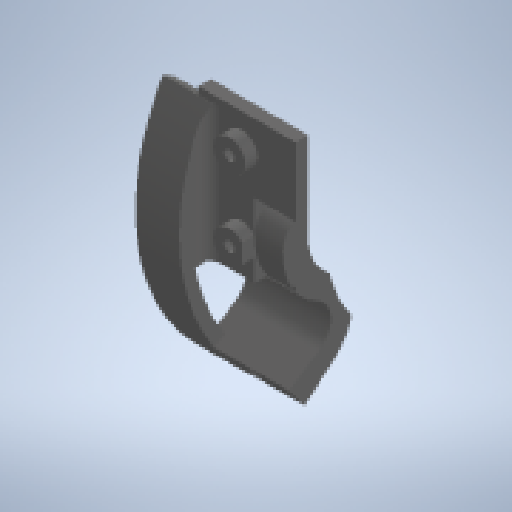
# Autodesk Inventor part: cover_back_right
Saved by Autodesk Inventor 2024.1 (Build 281209000, 209)
## iProperties
Created: 2025-01-10
Part Number: cover_back_right
Material: 一般
Document SubType Name: Modeling
Designer: hibik
Density: 1 g/cm^3
Appearance: 既定
Author: hibik
Autodesk Inventor part; units mm, degrees
ref_plane "YZ Plane" through (0, 0, 0) normal (1, 0, 0) x (0, 1, 0)
ref_plane "XZ Plane" through (0, 0, 0) normal (0, 1, 0) x (-1, 0, 0)
sketch "スケッチ1" plane through (0, 0, 0) normal (0, 0, 1) x (1, 0, 0)
  line L0 (10.5, 6.25) -> (-10.5, 6.25) construction
  line L1 (-10.5, 6.25) -> (-10.5, -6.25) construction
  line L2 (-10.5, -6.25) -> (10.5, -6.25) construction
  line L3 (10.5, -6.25) -> (10.5, 6.25) construction
  line L4 (10.5, 6.25) -> (-10.5, -6.25) construction
  line L5 (-10.5, 6.25) -> (10.5, -6.25) construction
  line L6 (-15.9, 11.28) -> (-2, 11.28)
  line L7 (-2, 11.28) -> (-2, -11.28)
  line L8 (-2, -11.28) -> (-15.9, -11.28)
  line L9 (-15.9, -11.28) -> (-15.9, 11.28)
  circle A0 centre (-10.5, 6.25) radius 0.85
  circle A1 centre (-10.5, -6.25) radius 0.85
  point P0 (0, 0)
  dimension "d0" = 21
  dimension "d1" = 12.5
  dimension "d2" = 2
  dimension "d3" = 15.9
  dimension "d4" = 5.03
  dimension "d5" = 5.03
  dimension "d7" = 1.7
  dimension "d8" = 1.7
  constraints: 20 end point, 4 parallel, 2 centre point, 2 coincident, 2 horizontal, 2 midpoint, 2 perpendicular
  measures "d0" distance of L0.start L0.end
  measures "d1" distance of L0.end L1.end
  measures "d2" distance from line of point (0, 0) L7
  measures "d3" distance from line of point (0, 0) L9
  measures "d4" distance between parallel lines of L6 L0
  measures "d5" distance between parallel lines of L8 L2
  measures "d7" diameter of A0
  measures "d8" diameter of A1
extrude "押し出し1" add sketch "スケッチ1" along normal blind 2
sketch "スケッチ2" plane through (0, 0, 2) normal (0, 0, 1) x (1, 0, 0)
  circle A0 centre (-10.5, 6.25) radius 0.85 projected
  circle A1 centre (-10.5, -6.25) radius 0.85 projected
  circle A2 centre (-10.5, 6.25) radius 2.5
  circle A3 centre (-10.5, -6.25) radius 2.5
  point P0 (0, 0)
  dimension "d11" = 5
  dimension "d12" = 5
  constraints: 2 centre point, 2 coincident
  measures "d11" diameter of A2
  measures "d12" diameter of A3
extrude "押し出し2" add sketch "スケッチ2" along normal blind 2
sketch "スケッチ3" plane through (-15.9, -11.28, 0) normal (-1, 0, 0) x (0, 0, 1)
  circle A0 centre (-26.25, 5.08) radius 26.25
  circle A1 centre (-26.25, 5.08) radius 30.75
  circle A2 centre (-26.25, 5.08) radius 32.75
  line L0 (6.5, 30) -> (6.5, 0) construction
  line L1 (4, 15.03) -> (4, 20.03) projected
  line L2 (-26.25, 5.08) -> (2.1123, 21.455)
  line L3 (-26.25, 5.08) -> (-9.875, -23.2823)
  line L4 (0, 22.56) -> (0, 0) projected
  line L5 (4, 18.38) -> (4, 16.68) projected
  line L6 (-72.1, 11.28) -> (19.6, 11.28) projected
  point P0 (0, 11.28)
  point P1 (0, 5.08)
  point P2 (0.3803, 20.455)
  point P3 (-10.875, -21.5503)
  point P4 (4, 17.53)
  dimension "d15" = 52.5
  dimension "d16" = 2.5
  dimension "d17" = 2
  dimension "d18" = 90
  dimension "d36" = 12.45
  dimension "d37" = 30
  constraints: 6 end point, 3 centre point, 2 coincident, 2 point on circle, 2 tangent, 1 horizontal alignment, 1 midpoint, 1 vertical
  measures "d15" diameter of A0
  measures "d16" distance between parallel lines of L1 L0
  measures "d17" radial gap between concentric circles of A2 A1
  measures "d18" angle of L3 L2
  measures "d36" vertical distance of point (4, 17.53) A0.centre
  measures "d37" angle of L6 L2
extrude "押し出し3" add sketch "スケッチ3" along normal blind 7 contours A1 L6 A2 L3 | A1 L2 A2 L6 picked at (5.3708, 0.6792) picked at (4.1065, 13.0583)
sketch "スケッチ5" plane through (0, 0, 0) normal (0, 0, -1) x (-1, 0, 0)
  line L0 (2, -11.28) -> (2, 11.28) projected
  line L1 (15.9, -11.28) -> (2, -11.28) projected
  line L2 (2, -4.75) -> (8.5, -4.75)
  line L3 (8.5, -4.75) -> (8.5, -11.28)
  line L4 (8.5, -11.28) -> (2, -11.28)
  line L5 (2, -11.28) -> (2, -4.75)
  line L6 (2, 11.28) -> (15.9, 11.28) projected
  circle A0 centre (10.5, 6.25) radius 0.85 projected
  circle A1 centre (10.5, -6.25) radius 2
  circle A2 centre (10.5, -6.25) radius 0.85 projected
  point P0 (0, 0)
  dimension "d26" = 11
  dimension "d27" = 4
  constraints: 8 end point, 2 parallel, 2 point on line, 1 centre point, 1 concentric, 1 horizontal, 1 perpendicular, 1 tangent
  measures "d26" distance from line of L2 A0.centre
  measures "d27" diameter of A1
extrude "押し出し5" cut sketch "スケッチ5" against normal through all contours L0 L2 L3 L1
sketch "スケッチ6" plane through (-2, 11.28, 2) normal (1, 0, 0) x (0, 0, -1)
  circle A0 centre (4, -16.03) radius 4
  line L0 (0, -16.03) -> (0, 0) projected
  line L1 (0, -16.03) -> (2, -16.03) projected
  line L2 (2, -16.03) -> (2, 0) projected
  line L3 (2, 0) -> (0, 0) projected
  line L4 (0, -16.03) -> (0, 0) projected
  circle A1 centre (4, -16.03) radius 6.5
  point P0 (2, -11.28)
  point P1 (2, -9.8453)
  point P2 (0, -10.9065)
  point P3 (0, -16.03)
  point P4 (2, -12.5659)
  dimension "d30" = 8
  dimension "d31" = 13
  constraints: 2 centre point, 1 coincident, 1 horizontal alignment, 1 tangent
  measures "d30" diameter of A0
  measures "d31" diameter of A1
extrude "押し出し6" cut sketch "スケッチ6" against normal up to surface (6.5 mm away) contours L0 A1 L2 A0 picked at (1.1078, -12.1766)
sketch "スケッチ7" plane through (-2, -4.75, 0) normal (1, 0, 0) x (0, 0, -1)
  circle A0 centre (2, 0) radius 4
  arc A1 (0, 3.4641) -> (-2, 0) centre (2, 0) ccw projected
  line L0 (-2, 0) -> (0, 0) projected
  line L1 (-2, 0) -> (6, 0)
  line L2 (2, 0) -> (2, 4)
  point P0 (0, 4.75)
  point P1 (-2, 0)
  constraints: 4 end point, 2 concentric, 2 point on circle, 1 centre point, 1 midpoint, 1 vertical
extrude "押し出し7" add sketch "スケッチ7" against normal up to surface (13.9 mm away) contours L2 L1 L0 A0
sketch "スケッチ8" plane through (-15.9, 11.28, 0) normal (-1, 0, 0) x (0, 0, 1)
  line L0 (2.1123, -1.105) -> (0.3803, -2.105) projected
  arc A0 (-10.875, -44.1103) -> (0.3803, -2.105) centre (-26.25, -17.48) ccw projected
  line L1 (-10.875, -44.1103) -> (-9.875, -45.8423) projected
  arc A1 (-9.875, -45.8423) -> (2.1123, -1.105) centre (-26.25, -17.48) ccw projected
  line L2 (0, -22.56) -> (2, -22.56) projected
  line L3 (0, -22.56) -> (-26.25, -17.48) construction
  line L4 (0, -22.56) -> (3.9399, -23.3225)
  line L5 (2, -5.335) -> (2, -22.56) projected
  arc A2 (2, -5.335) -> (0.3803, -2.105) centre (-26.25, -17.48) ccw projected
  line L6 (0.3803, -2.105) -> (2, -1.1699) projected
  line L7 (2, 0) -> (2, -1.1699) projected
  line L8 (0, 0) -> (2, 0) projected
  line L9 (0, 0) -> (0, -12.5659) projected
  arc A3 (0, -12.5659) -> (-2, -12.03) centre (-2, -16.03) ccw projected
  line L10 (-2, -16.03) -> (-2, -12.03) projected
  line L11 (0, -16.03) -> (-2, -16.03) projected
  line L12 (0, -16.03) -> (0, -22.56) projected
  line L13 (0, -22.56) -> (2, -22.56) projected
  point P0 (0, -11.28)
  point P1 (2, -1.1699)
  constraints: 4 end point, 1 coincident, 1 collinear, 1 point on circle
extrude "押し出し8" add sketch "スケッチ8" along normal blind 1.5 contours L0 A0 L5 L2 L12 L11 L10 A3 L9 L8 L7 | A0 L4 L2 L5
fillet "フィレット1" radius 2 2 edges at (-15.9, -2.6675, 2) (-15.9, 8.0276, 2)
fillet "フィレット2" radius 2 1 edges at (-5.25, -1.2859, 0)
sketch "スケッチ11" plane through (-2, -4.75, -2) normal (1, 0, 0) x (0, 0, -1)
  arc A0 (-4.6, -13) -> (1.3476, -9.3399) centre (-0.5, -13) ccw projected
  arc A1 (-4.4, 0) -> (1.3476, -9.3399) centre (6.0625, 0) ccw projected
  line L0 (-6, -3) -> (-6, 0) projected
  line L1 (-4, -3) -> (-6, -3) projected
  line L2 (-4, -6.53) -> (-4, -3) projected
  line L3 (-2, 0) -> (-4, 0) projected
  line L4 (-6, 0) -> (-4, 0) projected
  arc A2 (0, 4) -> (-4, 0) centre (0, 0) ccw projected
  line L5 (-4, 0) -> (0, 0) projected
  line L6 (0, 0) -> (0, 4) projected
  arc A3 (-4, 0) -> (-2.112, -6.53) centre (8.2368, 0) ccw
  arc A4 (0, 4) -> (-4, 0) centre (0, 0) ccw projected
  line L7 (-6, -3) -> (-6, 0) projected
  line L8 (-4, -3) -> (-6, -3) projected
  line L9 (-4, -6.53) -> (-4, -3) projected
  line L10 (-2, -6.53) -> (-4, -6.53) projected
  line L11 (-2, 0) -> (-2, -6.53) projected
  line L12 (-2, 0) -> (-4, 0) projected
  line L13 (-6, 0) -> (-4, 0) projected
  arc A5 (0, 0) -> (7.6451, -8.2155) centre (8.2368, 0) ccw
  circle A6 centre (-0.5, -13) radius 7.4263
  line L14 (-2, -6.53) -> (-6, -6.53) projected
  line L15 (-6, 11.0999) -> (-6, -6.53) projected
  arc A7 (-6, 11.0999) -> (7.875, -29.8123) centre (24.25, -1.45) ccw projected
  line L16 (8.875, -28.0803) -> (7.875, -29.8123) projected
  arc A8 (-5.9399, -7.2925) -> (8.875, -28.0803) centre (24.25, -1.45) ccw projected
  line L17 (-2, -6.53) -> (-5.9399, -7.2925) projected
  line L18 (-4, -14.0481) -> (-6.1965, -14.0481) projected
  line L19 (-4, -14.0481) -> (-3.8009, -14.0481)
  line L20 (-3.0122, -19.5976) -> (24.25, -1.45)
  line L21 (-0.5437, -22.8471) -> (24.25, -1.45)
  point P0 (-2, 4.75)
  point P1 (-2.5105, -5.8511)
  point P2 (-2, -5.7268)
  point P3 (-2.097, -6.5488)
  point P4 (1.7719, -16.413)
  point P5 (4.3519, -18.6221)
  point P6 (3.6423, -6.8364)
  constraints: 8 point on circle, 6 end point, 4 tangent, 3 centre point, 2 coincident, 2 point on line, 1 concentric
extrude "押し出し10" add sketch "スケッチ11" against normal up to surface (15.4 mm away) contours L20 A6 A8 | A0 A1 L17 L11 A6 L20 | A8 A6 A7 L20 | A8 L21 A7 A6 | A6 L21 A8 | A6 L11 L5 A5 | A6 A3 L3 L11
ref_plane "作業平面1" through (-2, -27.5971, -1.4563) normal (0, -0.6533458, 0.7570597) x (1, 0, 0)
sketch "スケッチ13" plane through (-2, -27.5971, -1.4563) normal (0, -0.6533458, 0.7570597) x (1, 0, 0)
  ellipse E0 centre (-8.5, 30.8225) end of major axis (-11.25, 30.8225) minor radius 2.0819 projected
  circle A0 centre (-8.5, 2.0364) radius 0.9
  line L0 (0, 0) -> (0, 4.0728) projected
  point P0 (2, 21.8441)
  point P1 (0, 2.0364)
  dimension "d48" = 1.8
  constraints: 1 centre point, 1 horizontal alignment, 1 midpoint, 1 vertical alignment, 1 other
  measures "d48" diameter of A0
extrude "押し出し11" cut sketch "スケッチ13" against normal blind 5 contours A0
sketch "スケッチ14" plane through (0, 0, 4) normal (0, 0, 1) x (1, 0, 0)
  circle A0 centre (-10.5, -6.25) radius 0.85 projected
  point P0 (0, 0)
extrude "押し出し12" cut sketch "スケッチ14" against normal through all
sketch "スケッチ15" plane through (-2, -4.75, -2) normal (1, 0, 0) x (0, 0, -1)
  arc A0 (0, 4) -> (-4, 0) centre (0, 0) ccw projected
  arc A1 (-4, 0) -> (-2.5105, -5.8511) centre (8.2368, 0) ccw projected
  arc A2 (-2, -5.7268) -> (-2.5105, -5.8511) centre (-0.5, -13) ccw projected
  line L0 (-2, -5.7268) -> (-2, -6.53) projected
  line L1 (-2, -6.53) -> (-2.097, -6.5488) projected
  arc A3 (-2.097, -6.5488) -> (1.3476, -9.3399) centre (6.0625, 0) ccw projected
  arc A4 (1.7719, -16.413) -> (1.3476, -9.3399) centre (-0.5, -13) ccw projected
  line L2 (1.7719, -16.413) -> (-3.0122, -19.5976) projected
  arc A5 (-3.0122, -19.5976) -> (-0.5437, -22.8471) centre (24.25, -1.45) ccw projected
  line L3 (-0.5437, -22.8471) -> (4.3519, -18.6221) projected
  arc A6 (4.3519, -18.6221) -> (3.6423, -6.8364) centre (-0.5, -13) ccw projected
  arc A7 (0, 0) -> (3.6423, -6.8364) centre (8.2368, 0) ccw projected
  line L4 (0, 0) -> (0, 4) projected
  point P0 (-2, 4.75)
extrude "押し出し13" cut sketch "スケッチ15" against normal blind 2
sketch "スケッチ16" plane through (-4, -4.75, -2) normal (1, 0, 0) x (0, 0, -1)
  arc A0 (3.3909, -6.6605) -> (6.8479, -14.076) centre (24.25, -1.45) ccw
  arc A1 (0, 4) -> (-4, 0) centre (0, 0) ccw projected
  arc A2 (-4, 0) -> (-2.5105, -5.8511) centre (8.2368, 0) ccw projected
  arc A3 (-2, -5.7268) -> (-2.5105, -5.8511) centre (-0.5, -13) ccw projected
  line L0 (-2, -6.53) -> (-2, -5.7268) projected
  line L1 (-2.097, -6.5488) -> (-2, -6.53) projected
  arc A4 (-2.097, -6.5488) -> (1.3476, -9.3399) centre (6.0625, 0) ccw projected
  arc A5 (1.7719, -16.413) -> (1.3476, -9.3399) centre (-0.5, -13) ccw projected
  line L2 (-3.0122, -19.5976) -> (1.7719, -16.413) projected
  arc A6 (-3.0122, -19.5976) -> (-0.5437, -22.8471) centre (24.25, -1.45) ccw projected
  line L3 (4.3519, -18.6221) -> (-0.5437, -22.8471) projected
  arc A7 (4.3519, -18.6221) -> (3.6423, -6.8364) centre (-0.5, -13) ccw projected
  arc A8 (0, 0) -> (3.6423, -6.8364) centre (8.2368, 0) ccw projected
  line L4 (0, 4) -> (0, 0) projected
  point P0 (-2, 4.75)
  point P1 (3.3909, -6.6605)
  point P2 (6.8479, -14.076)
  constraints: 2 point on circle, 1 centre point, 4 other
extrude "押し出し14" cut sketch "スケッチ16" against normal through all contours A8 A7 A0
equation "\"d5\" = d4"
